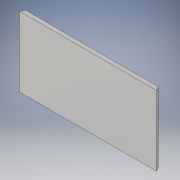
# Autodesk Inventor part: Side Wall
Saved by Autodesk Inventor 2017 (Build 210142000, 142)
## iProperties
Created: 2017-06-10
Part Number: Side Wall
Material: Generic
Document SubType Name: Modeling
Designer: Matthew
Density: 1 g/cm^3
Appearance: Aluminum - Polished
Author: Matthew
Autodesk Inventor part; units mm, degrees
ref_plane "YZ Plane" through (0, 0, 0) normal (1, 0, 0) x (0, 1, 0)
ref_plane "XZ Plane" through (0, 0, 0) normal (0, 1, 0) x (-1, 0, 0)
ref_plane "XY Plane" through (0, 0, 0) normal (0, 0, 1) x (1, 0, 0)
sketch "Sketch1" plane through (0, 0, 0) normal (0, 1, 0) x (-1, 0, 0)
  line L0 (0, 0) -> (105.6851, 0)
  line L1 (105.6851, 0) -> (105.6851, -3.175)
  line L2 (105.6851, -3.175) -> (0, -3.175)
  line L3 (0, -3.175) -> (0, 0)
  dimension "d0" = 3.175
  dimension "d1" = 105.6851
  constraints: 8 end point, 2 parallel, 1 horizontal, 1 perpendicular
  measures "d0" distance of L2.end L0.start
  measures "d1" distance of L0.start L0.end
extrude "Extrusion1" add sketch "Sketch1" along normal blind 53.975
sketch "Sketch2" plane through (0, 53.975, 0) normal (0, 1, 0) x (1, 0, 0)
  line L0 (-105.6851, 3.175) -> (-105.6851, 0) projected
  line L1 (-105.6851, 0) -> (-99.7525, 10.8664)
  line L2 (-105.6851, 0) -> (0, 0) projected
  line L3 (0, 0) -> (-13.3627, 24.476)
  line L4 (0, 3.175) -> (-105.6851, 3.175) projected
  line L5 (-1.7334, 3.175) -> (0, 3.175)
  line L6 (0, 3.175) -> (0, 0)
  line L7 (-103.9517, 3.175) -> (-105.6851, 3.175)
  line L8 (-105.6851, 0) -> (-105.6851, 3.175)
  dimension "d4" = 61.368
  dimension "d5" = 61.368
  constraints: 12 end point, 4 point on line, 3 collinear, 1 perpendicular
  measures "d4" angle of L2 L1
  measures "d5" angle of L2 L3
extrude "Extrusion2" cut sketch "Sketch2" against normal blind 53.975 contours L4 L1 L0 | L3 L4 L6
body "Solid1"
